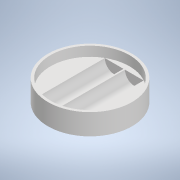
# Autodesk Inventor part: EnclosureBase
Saved by Autodesk Inventor 2020 (Build 240168000, 168)
## iProperties
Created: 2020-10-17
Part Number: EnclosureBase
Material: Generic
Document SubType Name: Modeling
Designer: vmiguel
Density: 1 g/cm^3
Appearance: Default
Author: vmiguel
Autodesk Inventor part; units mm, degrees
ref_plane "YZ Plane" through (0, 0, 0) normal (1, 0, 0) x (0, 1, 0)
ref_plane "XZ Plane" through (0, 0, 0) normal (0, 1, 0) x (-1, 0, 0)
ref_plane "XY Plane" through (0, 0, 0) normal (0, 0, 1) x (1, 0, 0)
sketch "Sketch1" plane through (0, 0, 0) normal (0, 1, 0) x (-1, 0, 0)
  circle A0 centre (0, 0) radius 50
  dimension "d0" = 100
  constraints: 1 centre point, 1 coincident
  measures "d0" diameter of A0
extrude "Extrusion1" add sketch "Sketch1" along normal blind 25
sketch "Sketch2" plane through (0, 0, 0) normal (0, -1, 0) x (1, 0, 0)
  circle A0 centre (0, 0) radius 25.25
  dimension "d3" = 50.5
  constraints: 1 centre point, 1 coincident
  measures "d3" diameter of A0
extrude "Extrusion2" cut sketch "Sketch2" against normal blind 0.4
sketch "Sketch3" plane through (0, 25, 0) normal (0, 1, 0) x (1, 0, 0)
  circle A0 centre (0, 0) radius 47
  circle A1 centre (0, 0) radius 50 projected
  dimension "d6" = 3
  constraints: 1 centre point, 1 coincident
  measures "d6" radial gap between concentric circles of A1 A0
extrude "Extrusion3" cut sketch "Sketch3" against normal blind 11.5 contours A0
sketch "Sketch5" plane through (0, 0, 0) normal (0, 0, 1) x (1, 0, 0)
  line L0 (-47, 13.5) -> (47, 13.5) construction
  circle A0 centre (12, 13.5) radius 11.125
  circle A1 centre (-12, 13.5) radius 11.125
  line L1 (0, 30.15) -> (0, -5.025) construction
  point P0 (0, 0)
  dimension "d9" = 22.25
  dimension "d10" = 22.25
  dimension "d11" = 12
  dimension "d12" = 12
  constraints: 2 centre point, 2 point on line
  measures "d9" diameter of A0
  measures "d10" diameter of A1
  measures "d11" distance from line of L1 A0.centre
  measures "d12" distance from line of A1.centre L1
extrude "Extrusion4" cut sketch "Sketch5" against normal mid plane 81.5
sketch "Sketch6" plane through (0, 0, 0) normal (0, -1, 0) x (1, 0, 0)
  line L0 (-30.5879, 38.6446) -> (30.5879, 38.6446) construction
  line L1 (30.5879, 38.6446) -> (30.5879, 30) construction
  line L2 (30.5879, 30) -> (-30.5879, 30) construction
  line L3 (-30.5879, 30) -> (-30.5879, 38.6446) construction
  circle A0 centre (0, 0) radius 25.25 projected
  spline S0 degree 2 poles (-20.901, 30.524) (-20.0192, 31.1693) (-19.1182, 33.8658) knots 0 0 0 1 1 1
  spline S1 degree 2 poles (-19.1182, 33.8658) (-18.6006, 35.4313) (-18.3962, 36.6965) knots 0 0 0 1 1 1
  spline S2 degree 2 poles (-18.3962, 36.6965) (-18.3387, 37.0479) (-18.3387, 37.2396) knots 0 0 0 1 1 1
  spline S3 degree 2 poles (-18.3387, 37.2396) (-18.5495, 37.2268) (-18.7284, 37.1246) knots 0 0 0 1 1 1
  line L4 (-18.7284, 37.1246) -> (-19.1118, 36.9073)
  spline S4 degree 2 poles (-19.1118, 36.9073) (-19.2652, 36.8179) (-19.7955, 37.2652) (-19.7508, 37.5783) (-19.4441, 37.7764) (-19.246, 37.853) knots 0 0 0 1 2 3 4 4 4
  spline S5 degree 2 poles (-19.246, 37.853) (-18.8307, 38) (-18.262, 38) (-17.8275, 37.9105) (-17.6486, 37.8083) knots 0 0 0 1 2 3 3 3
  spline S6 degree 2 poles (-17.6486, 37.8083) (-17.2396, 37.5719) (-17.2268, 37.1374) knots 0 0 0 1 1 1
  spline S7 degree 2 poles (-17.2268, 37.1374) (-17.2077, 36.3706) (-17.7444, 34.5495) knots 0 0 0 1 1 1
  spline S8 degree 2 poles (-17.7444, 34.5495) (-18.5942, 31.6613) (-19.738, 30.492) knots 0 0 0 1 1 1
  spline S9 degree 2 poles (-19.738, 30.492) (-20.0511, 30.1661) (-20.3898, 30.0511) knots 0 0 0 1 1 1
  spline S10 degree 2 poles (-20.3898, 30.0511) (-20.4792, 30.0128) (-20.6709, 30.0128) (-20.8243, 30.0831) (-20.8754, 30.1342) knots 0 0 0 1 2 3 3 3
  spline S11 degree 2 poles (-20.8754, 30.1342) (-20.9776, 30.23) (-20.9776, 30.4665) (-20.901, 30.524) knots 0 0 0 1 2 2 2
  spline S12 degree 2 poles (-13.6358, 30.8051) (-13.7444, 31.0927) (-13.7188, 31.9042) (-13.5144, 33.0479) (-13.2971, 33.7061) knots 0 0 0 1 2 3 3 3
  spline S13 degree 2 poles (-13.2971, 33.7061) (-12.7987, 35.2204) (-11.9489, 36.3898) knots 0 0 0 1 1 1
  spline S14 degree 2 poles (-11.9489, 36.3898) (-11.8019, 36.5879) (-11.476, 36.5879) (-11.1693, 36.4473) (-11.0479, 36.345) knots 0 0 0 1 2 3 3 3
  spline S15 degree 2 poles (-11.0479, 36.345) (-10.754, 36.1022) (-10.8562, 35.9489) knots 0 0 0 1 1 1
  spline S16 degree 2 poles (-10.8562, 35.9489) (-11.5719, 34.7923) (-12.0319, 33.8658) knots 0 0 0 1 1 1
  spline S17 degree 2 poles (-12.0319, 33.8658) (-10.8754, 33.9425) (-9.9936, 34.6006) knots 0 0 0 1 1 1
  spline S18 degree 2 poles (-9.9936, 34.6006) (-9.0224, 35.3099) (-9.0224, 36.3259) knots 0 0 0 1 1 1
  spline S19 degree 2 poles (-9.0224, 36.3259) (-9.0224, 37.016) (-9.7125, 37.2077) knots 0 0 0 1 1 1
  spline S20 degree 2 poles (-9.7125, 37.2077) (-9.9169, 37.2652) (-10.4984, 37.2652) (-11.1182, 37.1438) (-11.3994, 37.0415) knots 0 0 0 1 2 3 3 3
  spline S21 degree 2 poles (-11.3994, 37.0415) (-11.9681, 36.8307) (-12.4409, 36.492) knots 0 0 0 1 1 1
  spline S22 degree 2 poles (-12.4409, 36.492) (-12.5687, 36.3962) (-12.7987, 36.3962) (-13.0607, 36.5112) (-13.1629, 36.6006) knots 0 0 0 1 2 3 3 3
  spline S23 degree 2 poles (-13.1629, 36.6006) (-13.5655, 36.9329) (-13.0543, 37.2971) knots 0 0 0 1 1 1
  spline S24 degree 2 poles (-13.0543, 37.2971) (-12.3131, 37.8211) (-10.8626, 37.9744) knots 0 0 0 1 1 1
  spline S25 degree 2 poles (-10.8626, 37.9744) (-10.5942, 38) (-9.6869, 38) (-8.7412, 37.6997) (-8.4601, 37.4505) knots 0 0 0 1 2 3 3 3
  spline S26 degree 2 poles (-8.4601, 37.4505) (-7.9297, 36.984) (-7.9297, 36.1406) knots 0 0 0 1 1 1
  spline S27 degree 2 poles (-7.9297, 36.1406) (-7.9297, 35.3866) (-8.5304, 34.6518) knots 0 0 0 1 1 1
  spline S28 degree 2 poles (-8.5304, 34.6518) (-9.0735, 33.9681) (-9.9425, 33.5463) knots 0 0 0 1 1 1
  spline S29 degree 2 poles (-9.9425, 33.5463) (-9.5272, 33.361) (-9.1118, 32.7029) (-9.131, 31.9425) (-9.4121, 31.3035) (-9.8914, 30.7859) (-10.5176, 30.3962) (-10.8626, 30.2684) knots 0 0 0 1 2 3 4 5 6 6 6
  spline S30 degree 2 poles (-10.8626, 30.2684) (-11.5719, 30) (-12.3067, 30) knots 0 0 0 1 1 1
  spline S31 degree 2 poles (-12.3067, 30) (-13.3355, 30) (-13.6358, 30.8051) knots 0 0 0 1 1 1
  spline S32 degree 2 poles (-12.3962, 33.0351) (-12.7859, 32.0703) (-12.8051, 31.3546) knots 0 0 0 1 1 1
  spline S33 degree 2 poles (-12.8051, 31.3546) (-12.8179, 31.0096) (-12.4537, 30.6326) (-11.8211, 30.6326) (-11.1438, 30.9073) (-10.8626, 31.1438) knots 0 0 0 1 2 3 4 4 4
  spline S34 degree 2 poles (-10.8626, 31.1438) (-10.2236, 31.6869) (-10.1981, 32.3706) knots 0 0 0 1 1 1
  spline S35 degree 2 poles (-10.1981, 32.3706) (-10.1853, 32.9968) (-10.7604, 33.2204) knots 0 0 0 1 1 1
  spline S36 degree 2 poles (-10.7604, 33.2204) (-10.9393, 33.2843) (-11.1374, 33.3035) knots 0 0 0 1 1 1
  spline S37 degree 2 poles (-11.1374, 33.3035) (-11.3738, 33.2971) (-12.2364, 33.0735) (-12.3962, 33.0351) knots 0 0 0 1 2 2 2
  spline S38 degree 2 poles (-8.0192, 31.8403) (-8, 32.2875) (-7.7444, 33.099) (-7.3163, 33.8594) (-6.7412, 34.5367) (-6.4026, 34.7923) knots 0 0 0 1 2 3 4 4 4
  spline S39 degree 2 poles (-6.4026, 34.7923) (-5.6677, 35.3419) (-4.9265, 35.3419) knots 0 0 0 1 1 1
  spline S40 degree 2 poles (-4.9265, 35.3419) (-4.0511, 35.3419) (-3.7572, 34.6198) knots 0 0 0 1 1 1
  spline S41 degree 2 poles (-3.7572, 34.6198) (-3.655, 34.377) (-3.6677, 33.7061) (-3.9105, 33.1374) (-4.345, 32.6709) (-4.9457, 32.3067) (-5.2971, 32.1789) knots 0 0 0 1 2 3 4 5 5 5
  spline S42 degree 2 poles (-5.2971, 32.1789) (-6.0256, 31.9233) (-6.8498, 31.9105) knots 0 0 0 1 1 1
  spline S43 degree 2 poles (-6.8498, 31.9105) (-6.869, 31.8403) (-6.8818, 31.5527) (-6.8115, 31.2013) (-6.722, 31.0607) knots 0 0 0 1 2 3 3 3
  spline S44 degree 2 poles (-6.722, 31.0607) (-6.5367, 30.754) (-6.1917, 30.754) knots 0 0 0 1 1 1
  spline S45 degree 2 poles (-6.1917, 30.754) (-5.5974, 30.754) (-5.0351, 31.1054) knots 0 0 0 1 1 1
  spline S46 degree 2 poles (-5.0351, 31.1054) (-4.8371, 31.2204) (-4.5879, 31.4696) (-4.4026, 31.4696) (-4.2684, 31.2524) (-4.2684, 31.1118) knots 0 0 0 1 2 3 4 4 4
  spline S47 degree 2 poles (-4.2684, 31.1118) (-4.2684, 30.8435) (-4.4217, 30.6454) knots 0 0 0 1 1 1
  spline S48 degree 2 poles (-4.4217, 30.6454) (-5.0607, 30) (-6.3323, 30) knots 0 0 0 1 1 1
  spline S49 degree 2 poles (-6.3323, 30) (-7.0863, 30) (-7.5399, 30.4473) knots 0 0 0 1 1 1
  spline S50 degree 2 poles (-7.5399, 30.4473) (-8.0511, 30.9585) (-8.0192, 31.8403) knots 0 0 0 1 1 1
  spline S51 degree 2 poles (-5.0351, 34.6581) (-5.5719, 34.6581) (-6.0703, 33.9233) knots 0 0 0 1 1 1
  spline S52 degree 2 poles (-6.0703, 33.9233) (-6.4856, 33.2907) (-6.7412, 32.4217) knots 0 0 0 1 1 1
  spline S53 degree 2 poles (-6.7412, 32.4217) (-5.8914, 32.5112) (-5.2652, 33.099) knots 0 0 0 1 1 1
  spline S54 degree 2 poles (-5.2652, 33.099) (-4.6837, 33.6486) (-4.6837, 34.6581) (-5.0351, 34.6581) knots 0 0 0 1 2 2 2
  spline S55 degree 2 poles (-2.8818, 30.2556) (-3.0096, 30.3898) (-3.1693, 30.8051) (-3.1693, 31.3482) (-2.9201, 32.2684) (-2.722, 32.8562) knots 0 0 0 1 2 3 4 4 4
  line L5 (-2.722, 32.8562) -> (-2.2939, 34.1278)
  spline S56 degree 2 poles (-2.2939, 34.1278) (-1.3802, 36.7859) (-1.2396, 38.2364) knots 0 0 0 1 1 1
  spline S57 degree 2 poles (-1.2396, 38.2364) (-1.1885, 38.6645) (-0.8179, 38.6645) knots 0 0 0 1 1 1
  spline S58 degree 2 poles (-0.8179, 38.6645) (-0.5815, 38.6645) (-0.4281, 38.5559) knots 0 0 0 1 1 1
  spline S59 degree 2 poles (-0.4281, 38.5559) (-0.1342, 38.3323) (-0.1534, 37.7764) (-0.3259, 36.984) (-0.607, 36.0511) (-0.7796, 35.5272) knots 0 0 0 1 2 3 4 4 4
  line L6 (-0.7796, 35.5272) -> (-1.4888, 33.4569)
  spline S60 degree 2 poles (-1.4888, 33.4569) (-2.0958, 31.6869) (-2.0958, 31.1693) knots 0 0 0 1 1 1
  spline S61 degree 2 poles (-2.0958, 31.1693) (-2.0958, 30.8946) (-1.8722, 30.8946) knots 0 0 0 1 1 1
  spline S62 degree 2 poles (-1.8722, 30.8946) (-1.655, 30.8946) (-1.3035, 31.0799) (-1.2524, 31.0799) knots 0 0 0 1 2 2 2
  spline S63 degree 2 poles (-1.2524, 31.0799) (-1.1438, 31.0799) (-1.1438, 30.9712) knots 0 0 0 1 1 1
  spline S64 degree 2 poles (-1.1438, 30.9712) (-1.1438, 30.5176) (-1.6102, 30.2109) knots 0 0 0 1 1 1
  spline S65 degree 2 poles (-1.6102, 30.2109) (-1.9233, 30) (-2.4409, 30) (-2.754, 30.1214) (-2.8818, 30.2556) knots 0 0 0 1 2 3 3 3
  spline S66 degree 2 poles (1.508, 31.0096) (1.6358, 31.0096) (1.6358, 30.8307) knots 0 0 0 1 1 1
  spline S67 degree 2 poles (1.6358, 30.8307) (1.6358, 30.6006) (1.4313, 30.3578) knots 0 0 0 1 1 1
  spline S68 degree 2 poles (1.4313, 30.3578) (1.1246, 30) (0.607, 30) knots 0 0 0 1 1 1
  spline S69 degree 2 poles (0.607, 30) (0.0128, 30) (-0.2045, 30.4792) knots 0 0 0 1 1 1
  spline S70 degree 2 poles (-0.2045, 30.4792) (-0.2875, 30.6518) (-0.2875, 31.131) (-0.1214, 31.7188) (0.1278, 32.3642) (0.2812, 32.6965) knots 0 0 0 1 2 3 4 4 4
  line L7 (0.2812, 32.6965) -> (0.5495, 33.3419)
  spline S71 degree 2 poles (0.5495, 33.3419) (0.8435, 34.0639) (0.8435, 34.524) (0.7476, 34.6709) (0.6901, 34.7093) knots 0 0 0 1 2 3 3 3
  line L8 (0.6901, 34.7093) -> (0.5879, 34.7859)
  spline S72 degree 2 poles (0.5879, 34.7859) (0.5367, 34.8179) (0.5367, 34.9968) (0.6773, 35.1629) (0.7923, 35.2204) knots 0 0 0 1 2 3 3 3
  spline S73 degree 2 poles (0.7923, 35.2204) (1.0224, 35.3419) (1.3291, 35.3419) knots 0 0 0 1 1 1
  spline S74 degree 2 poles (1.3291, 35.3419) (2.0767, 35.3419) (2.0767, 34.9457) knots 0 0 0 1 1 1
  spline S75 degree 2 poles (2.0767, 34.9457) (2.0767, 34.4856) (1.5974, 33.3035) (1.4313, 32.9457) knots 0 0 0 1 2 2 2
  line L9 (1.4313, 32.9457) -> (1.1246, 32.2364)
  spline S76 degree 2 poles (1.1246, 32.2364) (0.7859, 31.4633) (0.7859, 31.1182) knots 0 0 0 1 1 1
  spline S77 degree 2 poles (0.7859, 31.1182) (0.7859, 30.8946) (1.0096, 30.8946) knots 0 0 0 1 1 1
  spline S78 degree 2 poles (1.0096, 30.8946) (1.2268, 30.8946) (1.4569, 31.0096) (1.508, 31.0096) knots 0 0 0 1 2 2 2
  spline S79 degree 2 poles (2.5495, 36.5367) (2.4409, 36.4217) (2.1534, 36.2684) (1.8403, 36.2364) (1.5591, 36.3706) (1.4569, 36.492) knots 0 0 0 1 2 3 4 4 4
  spline S80 degree 2 poles (1.4569, 36.492) (1.2332, 36.7476) (1.2332, 37.2652) (1.4058, 37.5272) (1.5335, 37.6102) knots 0 0 0 1 2 3 3 3
  spline S81 degree 2 poles (1.5335, 37.6102) (1.7764, 37.77) (2.2109, 37.77) (2.4473, 37.7061) (2.5495, 37.6358) knots 0 0 0 1 2 3 3 3
  spline S82 degree 2 poles (2.5495, 37.6358) (2.8051, 37.4696) (2.8051, 36.984) (2.6645, 36.6581) (2.5495, 36.5367) knots 0 0 0 1 2 3 3 3
  spline S83 degree 2 poles (2.8435, 31.8403) (2.8626, 32.2875) (3.1182, 33.099) (3.5463, 33.8594) (4.1214, 34.5367) (4.4601, 34.7923) knots 0 0 0 1 2 3 4 4 4
  spline S84 degree 2 poles (4.4601, 34.7923) (5.1949, 35.3419) (5.9361, 35.3419) knots 0 0 0 1 1 1
  spline S85 degree 2 poles (5.9361, 35.3419) (6.8115, 35.3419) (7.1054, 34.6198) knots 0 0 0 1 1 1
  spline S86 degree 2 poles (7.1054, 34.6198) (7.2077, 34.377) (7.1949, 33.7061) (6.9521, 33.1374) (6.5176, 32.6709) (5.9169, 32.3067) (5.5655, 32.1789) knots 0 0 0 1 2 3 4 5 5 5
  spline S87 degree 2 poles (5.5655, 32.1789) (4.8371, 31.9233) (4.0128, 31.9105) knots 0 0 0 1 1 1
  spline S88 degree 2 poles (4.0128, 31.9105) (3.9936, 31.8403) (3.9808, 31.5527) (4.0511, 31.2013) (4.1406, 31.0607) knots 0 0 0 1 2 3 3 3
  spline S89 degree 2 poles (4.1406, 31.0607) (4.3259, 30.754) (4.6709, 30.754) knots 0 0 0 1 1 1
  spline S90 degree 2 poles (4.6709, 30.754) (5.2652, 30.754) (5.8275, 31.1054) knots 0 0 0 1 1 1
  spline S91 degree 2 poles (5.8275, 31.1054) (6.0256, 31.2204) (6.2748, 31.4696) (6.4601, 31.4696) (6.5942, 31.2524) (6.5942, 31.1118) knots 0 0 0 1 2 3 4 4 4
  spline S92 degree 2 poles (6.5942, 31.1118) (6.5942, 30.8435) (6.4409, 30.6454) knots 0 0 0 1 1 1
  spline S93 degree 2 poles (6.4409, 30.6454) (5.8019, 30) (4.5304, 30) knots 0 0 0 1 1 1
  spline S94 degree 2 poles (4.5304, 30) (3.7764, 30) (3.3227, 30.4473) knots 0 0 0 1 1 1
  spline S95 degree 2 poles (3.3227, 30.4473) (2.8115, 30.9585) (2.8435, 31.8403) knots 0 0 0 1 1 1
  spline S96 degree 2 poles (5.8275, 34.6581) (5.2907, 34.6581) (4.7923, 33.9233) knots 0 0 0 1 1 1
  spline S97 degree 2 poles (4.7923, 33.9233) (4.377, 33.2907) (4.1214, 32.4217) knots 0 0 0 1 1 1
  spline S98 degree 2 poles (4.1214, 32.4217) (4.9712, 32.5112) (5.5974, 33.099) knots 0 0 0 1 1 1
  spline S99 degree 2 poles (5.5974, 33.099) (6.1789, 33.6486) (6.1789, 34.6581) (5.8275, 34.6581) knots 0 0 0 1 2 2 2
  spline S100 degree 2 poles (7.7508, 30.5495) (7.6741, 30.7157) (7.6741, 31.1757) (7.8147, 31.7316) (8.0383, 32.3131) (8.1789, 32.6198) knots 0 0 0 1 2 3 4 4 4
  line L10 (8.1789, 32.6198) -> (8.4409, 33.2077)
  spline S101 degree 2 poles (8.4409, 33.2077) (8.9457, 34.377) (8.8115, 34.5879) knots 0 0 0 1 1 1
  spline S102 degree 2 poles (8.8115, 34.5879) (8.754, 34.6837) (8.5751, 34.7859) knots 0 0 0 1 1 1
  spline S103 degree 2 poles (8.5751, 34.7859) (8.524, 34.8179) (8.524, 34.9968) (8.6709, 35.1629) (8.7923, 35.2204) knots 0 0 0 1 2 3 3 3
  spline S104 degree 2 poles (8.7923, 35.2204) (9.0351, 35.3419) (9.5399, 35.3419) (9.8019, 35.2332) (9.885, 35.1502) knots 0 0 0 1 2 3 3 3
  spline S105 degree 2 poles (9.885, 35.1502) (10.0511, 34.984) (10.0511, 34.5048) (9.8658, 33.8978) (9.5911, 33.2332) (9.4249, 32.8882) knots 0 0 0 1 2 3 4 4 4
  line L11 (9.4249, 32.8882) -> (9.1246, 32.2173)
  spline S106 degree 2 poles (9.1246, 32.2173) (8.8051, 31.476) (8.8051, 31.2396) knots 0 0 0 1 1 1
  spline S107 degree 2 poles (8.8051, 31.2396) (8.8051, 30.7668) (9.1374, 30.7668) knots 0 0 0 1 1 1
  spline S108 degree 2 poles (9.1374, 30.7668) (9.9872, 30.7668) (10.7348, 31.7764) knots 0 0 0 1 1 1
  spline S109 degree 2 poles (10.7348, 31.7764) (11.1693, 32.3642) (11.3546, 33.0543) knots 0 0 0 1 1 1
  spline S110 degree 2 poles (11.3546, 33.0543) (11.4441, 33.3802) (11.4441, 33.9169) (11.4058, 34.2748) (11.3674, 34.4153) knots 0 0 0 1 2 3 3 3
  spline S111 degree 2 poles (11.3674, 34.4153) (11.3035, 34.6581) (11.1438, 34.8371) knots 0 0 0 1 1 1
  spline S112 degree 2 poles (11.1438, 34.8371) (11.0351, 34.9712) (11.2396, 35.1502) knots 0 0 0 1 1 1
  spline S113 degree 2 poles (11.2396, 35.1502) (11.4633, 35.3419) (11.8786, 35.3419) knots 0 0 0 1 1 1
  spline S114 degree 2 poles (11.8786, 35.3419) (12.1342, 35.3419) (12.3259, 35.099) knots 0 0 0 1 1 1
  spline S115 degree 2 poles (12.3259, 35.099) (12.5751, 34.8115) (12.5751, 33.7444) (12.2556, 32.722) (11.7061, 31.7764) (10.9521, 30.9585) (10.5176, 30.6518) knots 0 0 0 1 2 3 4 5 5 5
  spline S116 degree 2 poles (10.5176, 30.6518) (9.5911, 30) (8.6581, 30) knots 0 0 0 1 1 1
  spline S117 degree 2 poles (8.6581, 30) (7.9872, 30) (7.7508, 30.5495) knots 0 0 0 1 1 1
  spline S118 degree 2 poles (13.131, 31.8403) (13.1502, 32.2875) (13.4058, 33.099) (13.8339, 33.8594) (14.4089, 34.5367) (14.7476, 34.7923) knots 0 0 0 1 2 3 4 4 4
  spline S119 degree 2 poles (14.7476, 34.7923) (15.4824, 35.3419) (16.2236, 35.3419) knots 0 0 0 1 1 1
  spline S120 degree 2 poles (16.2236, 35.3419) (17.099, 35.3419) (17.393, 34.6198) knots 0 0 0 1 1 1
  spline S121 degree 2 poles (17.393, 34.6198) (17.4952, 34.377) (17.4824, 33.7061) (17.2396, 33.1374) (16.8051, 32.6709) (16.2045, 32.3067) (15.853, 32.1789) knots 0 0 0 1 2 3 4 5 5 5
  spline S122 degree 2 poles (15.853, 32.1789) (15.1246, 31.9233) (14.3003, 31.9105) knots 0 0 0 1 1 1
  spline S123 degree 2 poles (14.3003, 31.9105) (14.2812, 31.8403) (14.2684, 31.5527) (14.3387, 31.2013) (14.4281, 31.0607) knots 0 0 0 1 2 3 3 3
  spline S124 degree 2 poles (14.4281, 31.0607) (14.6134, 30.754) (14.9585, 30.754) knots 0 0 0 1 1 1
  spline S125 degree 2 poles (14.9585, 30.754) (15.5527, 30.754) (16.115, 31.1054) knots 0 0 0 1 1 1
  spline S126 degree 2 poles (16.115, 31.1054) (16.3131, 31.2204) (16.5623, 31.4696) (16.7476, 31.4696) (16.8818, 31.2524) (16.8818, 31.1118) knots 0 0 0 1 2 3 4 4 4
  spline S127 degree 2 poles (16.8818, 31.1118) (16.8818, 30.8435) (16.7284, 30.6454) knots 0 0 0 1 1 1
  spline S128 degree 2 poles (16.7284, 30.6454) (16.0895, 30) (14.8179, 30) knots 0 0 0 1 1 1
  spline S129 degree 2 poles (14.8179, 30) (14.0639, 30) (13.6102, 30.4473) knots 0 0 0 1 1 1
  spline S130 degree 2 poles (13.6102, 30.4473) (13.099, 30.9585) (13.131, 31.8403) knots 0 0 0 1 1 1
  spline S131 degree 2 poles (16.115, 34.6581) (15.5783, 34.6581) (15.0799, 33.9233) knots 0 0 0 1 1 1
  spline S132 degree 2 poles (15.0799, 33.9233) (14.6645, 33.2907) (14.4089, 32.4217) knots 0 0 0 1 1 1
  spline S133 degree 2 poles (14.4089, 32.4217) (15.2588, 32.5112) (15.885, 33.099) knots 0 0 0 1 1 1
  spline S134 degree 2 poles (15.885, 33.099) (16.4665, 33.6486) (16.4665, 34.6581) (16.115, 34.6581) knots 0 0 0 1 2 2 2
  point P0 (0, 30)
  dimension "d17" = 30
  constraints: 1 midpoint, 1 vertical alignment, 2 other
  measures "d17" distance from line of point (0, 0) L2
emboss "Emboss1" sketch "Sketch6" operation cut depth 1.5 direction (0, 1, 0) contours S0 S1 S2 S3 L4 S4 S5 S6 S7 S8 S9 S10 S11 | S12 S13 S14 S15 S16 S17 S18 S19 S20 S21 S22 S23 S24 S25 S26 S27 S28 S29 S30 S31 | S38 S39 S40 S41 S42 S43 S44 S45 S46 S47 S48 S49 S50 | S55 L5 S56 S57 S58 S59 L6 S60 S61 S62 S63 S64 S65 | S66 S67 S68 S69 S70 L7 S71 L8 S72 S73 S74 S75 L9 S76 S77 S78 | S79 S80 S81 S82 | S83 S84 S85 S86 S87 S88 S89 S90 S91 S92 S93 S94 S95 | S100 L10 S101 S102 S103 S104 S105 L11 S106 S107 S108 S109 S110 S111 S112 S113 S114 S115 S116 S117 | S118 S119 S120 S121 S122 S123 S124 S125 S126 S127 S128 S129 S130
sketch "Sketch7" plane through (0, 13.5, 0) normal (0, 1, 0) x (1, 0, 0)
  line L0 (23.125, -24.5019) -> (23.125, 24.5019) construction
  line L1 (23.125, 24.5019) -> (33.125, 24.5019) construction
  line L2 (33.125, 24.5019) -> (33.125, -24.5019) construction
  line L3 (33.125, -24.5019) -> (23.125, -24.5019) construction
  line L4 (-23.125, -40.75) -> (-23.125, 40.75) projected
  line L5 (-33.125, -20.8949) -> (-33.125, 20.8949) construction
  line L6 (-33.125, 20.8949) -> (-23.125, 20.8949) construction
  line L7 (-23.125, 20.8949) -> (-23.125, -20.8949) construction
  line L8 (-23.125, -20.8949) -> (-33.125, -20.8949) construction
  line L9 (23.125, 40.75) -> (23.125, -40.75) projected
  spline S0 degree 2 poles (-25.387, -7.9808) (-25.6042, -8.0958) (-26.1026, -8.2045) (-26.6522, -8.2045) (-27.5467, -8.0192) (-28.5435, -7.6869) (-29.5851, -7.2524) (-30.0835, -7.0096) knots 0 0 0 1 2 3 4 5 6 6 6
  spline S1 degree 2 poles (-30.0835, -7.0096) (-31.1186, -6.5112) (-31.8726, -6.0128) knots 0 0 0 1 1 1
  line L10 (-31.8726, -6.0128) -> (-31.8726, -6.0703)
  spline S2 degree 2 poles (-31.8726, -6.0703) (-31.8726, -6.6773) (-31.5978, -7.2013) knots 0 0 0 1 1 1
  spline S3 degree 2 poles (-31.5978, -7.2013) (-31.502, -7.3291) (-31.502, -7.4441) knots 0 0 0 1 1 1
  spline S4 degree 2 poles (-31.502, -7.4441) (-31.502, -7.6869) (-31.7384, -7.9169) knots 0 0 0 1 1 1
  spline S5 degree 2 poles (-31.7384, -7.9169) (-32.3007, -8.4537) (-32.6713, -7.2843) knots 0 0 0 1 1 1
  spline S6 degree 2 poles (-32.6713, -7.2843) (-32.8502, -6.7412) (-32.8502, -6.0703) (-32.6394, -5.6613) (-32.4988, -5.5208) knots 0 0 0 1 2 3 3 3
  spline S7 degree 2 poles (-32.4988, -5.5208) (-32.2688, -5.2907) (-31.8343, -5.1054) (-31.502, -5.1054) (-30.9397, -5.3035) (-30.6266, -5.4569) knots 0 0 0 1 2 3 4 4 4
  line L11 (-30.6266, -5.4569) -> (-29.9493, -5.8019)
  spline S8 degree 2 poles (-29.9493, -5.8019) (-29.5978, -5.9872) (-28.8183, -6.3578) (-28.0451, -6.722) (-27.6745, -6.869) knots 0 0 0 1 2 3 3 3
  spline S9 degree 2 poles (-27.6745, -6.869) (-26.8566, -7.1757) (-26.2815, -7.1757) knots 0 0 0 1 1 1
  spline S10 degree 2 poles (-26.2815, -7.1757) (-25.9365, -7.1757) (-25.7065, -7.1118) knots 0 0 0 1 1 1
  spline S11 degree 2 poles (-25.7065, -7.1118) (-26.0643, -6.8882) (-26.4541, -6.5623) knots 0 0 0 1 1 1
  line L12 (-26.4541, -6.5623) -> (-27.2592, -5.8466)
  spline S12 degree 2 poles (-27.2592, -5.8466) (-28.5946, -4.6006) (-29.0355, -4.23) knots 0 0 0 1 1 1
  spline S13 degree 2 poles (-29.0355, -4.23) (-30.0643, -3.3546) (-30.9716, -2.8882) knots 0 0 0 1 1 1
  spline S14 degree 2 poles (-30.9716, -2.8882) (-31.3359, -2.7029) (-31.6298, -2.7029) knots 0 0 0 1 1 1
  spline S15 degree 2 poles (-31.6298, -2.7029) (-32.1793, -2.7029) (-32.4541, -3.0032) knots 0 0 0 1 1 1
  spline S16 degree 2 poles (-32.4541, -3.0032) (-32.5627, -3.1118) (-32.8694, -2.9521) (-32.9461, -2.869) knots 0 0 0 1 2 2 2
  spline S17 degree 2 poles (-32.9461, -2.869) (-33.125, -2.6709) (-33.125, -2.1725) (-32.9205, -1.8211) (-32.7608, -1.7125) knots 0 0 0 1 2 3 3 3
  spline S18 degree 2 poles (-32.7608, -1.7125) (-32.4477, -1.4952) (-31.5276, -1.4952) (-30.4924, -1.8914) (-29.5084, -2.5304) (-28.5819, -3.3419) (-28.1601, -3.7636) knots 0 0 0 1 2 3 4 5 5 5
  line L13 (-28.1601, -3.7636) -> (-26.7033, -5.3099)
  spline S19 degree 2 poles (-26.7033, -5.3099) (-26.0004, -6.0064) (-25.7384, -6.2428) knots 0 0 0 1 1 1
  spline S20 degree 2 poles (-25.7384, -6.2428) (-25.24, -6.6901) (-24.9205, -6.9457) (-24.863, -7.1502) (-24.863, -7.5016) (-25.1697, -7.8658) (-25.387, -7.9808) knots 0 0 0 1 2 3 4 5 5 5
  spline S21 degree 2 poles (-25.8598, -0.8243) (-25.8598, -0.6965) (-25.6809, -0.6965) knots 0 0 0 1 1 1
  spline S22 degree 2 poles (-25.6809, -0.6965) (-25.4509, -0.6965) (-25.2081, -0.901) knots 0 0 0 1 1 1
  spline S23 degree 2 poles (-25.2081, -0.901) (-24.8502, -1.2077) (-24.8502, -1.7252) knots 0 0 0 1 1 1
  spline S24 degree 2 poles (-24.8502, -1.7252) (-24.8502, -2.3195) (-25.3295, -2.5367) knots 0 0 0 1 1 1
  spline S25 degree 2 poles (-25.3295, -2.5367) (-25.502, -2.6198) (-25.9812, -2.6198) (-26.5691, -2.4537) (-27.2145, -2.2045) (-27.5467, -2.0511) knots 0 0 0 1 2 3 4 4 4
  line L14 (-27.5467, -2.0511) -> (-28.1921, -1.7827)
  spline S26 degree 2 poles (-28.1921, -1.7827) (-28.9141, -1.4888) (-29.3742, -1.4888) (-29.5212, -1.5847) (-29.5595, -1.6422) knots 0 0 0 1 2 3 3 3
  line L15 (-29.5595, -1.6422) -> (-29.6362, -1.7444)
  spline S27 degree 2 poles (-29.6362, -1.7444) (-29.6681, -1.7955) (-29.847, -1.7955) (-30.0132, -1.655) (-30.0707, -1.5399) knots 0 0 0 1 2 3 3 3
  spline S28 degree 2 poles (-30.0707, -1.5399) (-30.1921, -1.3099) (-30.1921, -1.0032) knots 0 0 0 1 1 1
  spline S29 degree 2 poles (-30.1921, -1.0032) (-30.1921, -0.2556) (-29.7959, -0.2556) knots 0 0 0 1 1 1
  spline S30 degree 2 poles (-29.7959, -0.2556) (-29.3359, -0.2556) (-28.1538, -0.7348) (-27.7959, -0.901) knots 0 0 0 1 2 2 2
  line L16 (-27.7959, -0.901) -> (-27.0867, -1.2077)
  spline S31 degree 2 poles (-27.0867, -1.2077) (-26.3135, -1.5463) (-25.9685, -1.5463) knots 0 0 0 1 1 1
  spline S32 degree 2 poles (-25.9685, -1.5463) (-25.7448, -1.5463) (-25.7448, -1.3227) knots 0 0 0 1 1 1
  spline S33 degree 2 poles (-25.7448, -1.3227) (-25.7448, -1.1054) (-25.8598, -0.8754) (-25.8598, -0.8243) knots 0 0 0 1 2 2 2
  spline S34 degree 2 poles (-31.387, 0.2173) (-31.272, 0.1086) (-31.1186, -0.1789) (-31.0867, -0.492) (-31.2208, -0.7732) (-31.3423, -0.8754) knots 0 0 0 1 2 3 4 4 4
  spline S35 degree 2 poles (-31.3423, -0.8754) (-31.5978, -1.099) (-32.1154, -1.099) (-32.3774, -0.9265) (-32.4605, -0.7987) knots 0 0 0 1 2 3 3 3
  spline S36 degree 2 poles (-32.4605, -0.7987) (-32.6202, -0.5559) (-32.6202, -0.1214) (-32.5563, 0.115) (-32.486, 0.2173) knots 0 0 0 1 2 3 3 3
  spline S37 degree 2 poles (-32.486, 0.2173) (-32.3199, 0.4728) (-31.8343, 0.4728) (-31.5084, 0.3323) (-31.387, 0.2173) knots 0 0 0 1 2 3 3 3
  spline S38 degree 2 poles (-29.2272, 4.1406) (-29.2272, 3.9808) (-28.6138, 3.3994) (-28.3646, 3.1885) knots 0 0 0 1 2 2 2
  line L17 (-28.3646, 3.1885) -> (-27.847, 2.754)
  line L18 (-27.847, 2.754) -> (-26.78, 1.9169)
  spline S39 degree 2 poles (-26.78, 1.9169) (-26.2177, 1.6166) (-25.8407, 1.4505) knots 0 0 0 1 1 1
  line L19 (-25.8407, 1.4505) -> (-25.2464, 1.1757)
  spline S40 degree 2 poles (-25.2464, 1.1757) (-25.0292, 1.0671) (-24.8502, 0.9073) (-24.8502, 0.639) (-24.9461, 0.3834) (-25.0228, 0.2939) knots 0 0 0 1 2 3 4 4 4
  spline S41 degree 2 poles (-25.0228, 0.2939) (-25.1889, 0.1022) (-25.3806, 0.1022) knots 0 0 0 1 1 1
  spline S42 degree 2 poles (-25.3806, 0.1022) (-25.4573, 0.1022) (-25.6809, 0.2109) knots 0 0 0 1 1 1
  line L20 (-25.6809, 0.2109) -> (-26.0962, 0.4089)
  spline S43 degree 2 poles (-26.0962, 0.4089) (-26.2815, 0.4984) (-26.5691, 0.6198) knots 0 0 0 1 1 1
  line L21 (-26.5691, 0.6198) -> (-27.2656, 0.9073)
  spline S44 degree 2 poles (-27.2656, 0.9073) (-28.7736, 1.508) (-29.2145, 1.508) knots 0 0 0 1 1 1
  spline S45 degree 2 poles (-29.2145, 1.508) (-29.4509, 1.508) (-29.5595, 1.3546) knots 0 0 0 1 1 1
  line L22 (-29.5595, 1.3546) -> (-29.6362, 1.2524)
  spline S46 degree 2 poles (-29.6362, 1.2524) (-29.6681, 1.2013) (-29.847, 1.2013) (-30.0132, 1.3419) (-30.0707, 1.4569) knots 0 0 0 1 2 3 3 3
  spline S47 degree 2 poles (-30.0707, 1.4569) (-30.1921, 1.6869) (-30.1921, 2.147) (-30.0899, 2.4026) (-30.0004, 2.492) knots 0 0 0 1 2 3 3 3
  spline S48 degree 2 poles (-30.0004, 2.492) (-29.8215, 2.6837) (-29.4317, 2.6837) (-29.0419, 2.5815) (-28.6394, 2.4345) (-28.2496, 2.2748) (-28.1026, 2.2045) knots 0 0 0 1 2 3 4 5 5 5
  line L23 (-28.1026, 2.2045) -> (-27.8854, 2.1022)
  spline S49 degree 2 poles (-27.8854, 2.1022) (-27.8023, 2.0639) (-27.8343, 2.0831) knots 0 0 0 1 1 1
  spline S50 degree 2 poles (-27.8343, 2.0831) (-28.6202, 2.6518) (-28.8438, 2.8307) knots 0 0 0 1 1 1
  line L24 (-28.8438, 2.8307) -> (-29.2784, 3.1885)
  spline S51 degree 2 poles (-29.2784, 3.1885) (-29.7384, 3.5783) (-29.8854, 3.8019) knots 0 0 0 1 1 1
  spline S52 degree 2 poles (-29.8854, 3.8019) (-30.1921, 4.262) (-30.1921, 4.7796) (-30.0579, 5.1374) (-29.9365, 5.2716) knots 0 0 0 1 2 3 3 3
  spline S53 degree 2 poles (-29.9365, 5.2716) (-29.6745, 5.5527) (-28.8694, 5.5527) (-27.9876, 5.1821) (-27.4445, 4.9137) (-27.1633, 4.7923) knots 0 0 0 1 2 3 4 4 4
  spline S54 degree 2 poles (-27.1633, 4.7923) (-26.3071, 4.4089) (-25.9173, 4.4089) knots 0 0 0 1 1 1
  spline S55 degree 2 poles (-25.9173, 4.4089) (-25.7448, 4.4089) (-25.7448, 4.6837) knots 0 0 0 1 1 1
  spline S56 degree 2 poles (-25.7448, 4.6837) (-25.7448, 4.901) (-25.9301, 5.2524) (-25.9301, 5.3035) knots 0 0 0 1 2 2 2
  spline S57 degree 2 poles (-25.9301, 5.3035) (-25.9301, 5.4121) (-25.8215, 5.4121) knots 0 0 0 1 1 1
  spline S58 degree 2 poles (-25.8215, 5.4121) (-25.3678, 5.4121) (-25.0611, 4.9457) knots 0 0 0 1 1 1
  spline S59 degree 2 poles (-25.0611, 4.9457) (-24.8502, 4.6326) (-24.8502, 4.1086) (-24.9653, 3.77) (-25.0867, 3.6358) knots 0 0 0 1 2 3 3 3
  spline S60 degree 2 poles (-25.0867, 3.6358) (-25.355, 3.3355) (-25.8407, 3.3355) knots 0 0 0 1 1 1
  spline S61 degree 2 poles (-25.8407, 3.3355) (-26.4349, 3.3355) (-27.3231, 3.7061) knots 0 0 0 1 1 1
  spline S62 degree 2 poles (-27.3231, 3.7061) (-27.9301, 3.9808) (-28.1538, 4.0895) knots 0 0 0 1 1 1
  line L25 (-28.1538, 4.0895) -> (-28.518, 4.262)
  spline S63 degree 2 poles (-28.518, 4.262) (-28.8438, 4.4217) (-29.2272, 4.4217) (-29.2272, 4.1406) knots 0 0 0 1 2 2 2
  spline S64 degree 2 poles (-25.8598, 8.0447) (-25.8598, 8.1725) (-25.6809, 8.1725) knots 0 0 0 1 1 1
  spline S65 degree 2 poles (-25.6809, 8.1725) (-25.4509, 8.1725) (-25.2081, 7.9681) knots 0 0 0 1 1 1
  spline S66 degree 2 poles (-25.2081, 7.9681) (-24.8502, 7.6613) (-24.8502, 7.1438) knots 0 0 0 1 1 1
  spline S67 degree 2 poles (-24.8502, 7.1438) (-24.8502, 6.5495) (-25.3295, 6.3323) knots 0 0 0 1 1 1
  spline S68 degree 2 poles (-25.3295, 6.3323) (-25.502, 6.2492) (-25.9812, 6.2492) (-26.5691, 6.4153) (-27.2145, 6.6645) (-27.5467, 6.8179) knots 0 0 0 1 2 3 4 4 4
  line L26 (-27.5467, 6.8179) -> (-28.1921, 7.0863)
  spline S69 degree 2 poles (-28.1921, 7.0863) (-28.9141, 7.3802) (-29.3742, 7.3802) (-29.5212, 7.2843) (-29.5595, 7.2268) knots 0 0 0 1 2 3 3 3
  line L27 (-29.5595, 7.2268) -> (-29.6362, 7.1246)
  spline S70 degree 2 poles (-29.6362, 7.1246) (-29.6681, 7.0735) (-29.847, 7.0735) (-30.0132, 7.2141) (-30.0707, 7.3291) knots 0 0 0 1 2 3 3 3
  spline S71 degree 2 poles (-30.0707, 7.3291) (-30.1921, 7.5591) (-30.1921, 7.8658) knots 0 0 0 1 1 1
  spline S72 degree 2 poles (-30.1921, 7.8658) (-30.1921, 8.6134) (-29.7959, 8.6134) knots 0 0 0 1 1 1
  spline S73 degree 2 poles (-29.7959, 8.6134) (-29.3359, 8.6134) (-28.1538, 8.1342) (-27.7959, 7.9681) knots 0 0 0 1 2 2 2
  line L28 (-27.7959, 7.9681) -> (-27.0867, 7.6613)
  spline S74 degree 2 poles (-27.0867, 7.6613) (-26.3135, 7.3227) (-25.9685, 7.3227) knots 0 0 0 1 1 1
  spline S75 degree 2 poles (-25.9685, 7.3227) (-25.7448, 7.3227) (-25.7448, 7.5463) knots 0 0 0 1 1 1
  spline S76 degree 2 poles (-25.7448, 7.5463) (-25.7448, 7.7636) (-25.8598, 7.9936) (-25.8598, 8.0447) knots 0 0 0 1 2 2 2
  spline S77 degree 2 poles (-31.387, 9.0863) (-31.272, 8.9776) (-31.1186, 8.6901) (-31.0867, 8.377) (-31.2208, 8.0958) (-31.3423, 7.9936) knots 0 0 0 1 2 3 4 4 4
  spline S78 degree 2 poles (-31.3423, 7.9936) (-31.5978, 7.77) (-32.1154, 7.77) (-32.3774, 7.9425) (-32.4605, 8.0703) knots 0 0 0 1 2 3 3 3
  spline S79 degree 2 poles (-32.4605, 8.0703) (-32.6202, 8.3131) (-32.6202, 8.7476) (-32.5563, 8.984) (-32.486, 9.0863) knots 0 0 0 1 2 3 3 3
  spline S80 degree 2 poles (-32.486, 9.0863) (-32.3199, 9.3419) (-31.8343, 9.3419) (-31.5084, 9.2013) (-31.387, 9.0863) knots 0 0 0 1 2 3 3 3
  spline S81 degree 2 poles (32.3199, -17.5687) (32.0323, -17.6773) (31.2208, -17.6518) (30.0771, -17.4473) (29.4189, -17.23) knots 0 0 0 1 2 3 3 3
  spline S82 degree 2 poles (29.4189, -17.23) (27.9046, -16.7316) (26.7352, -15.8818) knots 0 0 0 1 1 1
  spline S83 degree 2 poles (26.7352, -15.8818) (26.5371, -15.7348) (26.5371, -15.4089) (26.6777, -15.1022) (26.78, -14.9808) knots 0 0 0 1 2 3 3 3
  spline S84 degree 2 poles (26.78, -14.9808) (27.0228, -14.6869) (27.1761, -14.7891) knots 0 0 0 1 1 1
  spline S85 degree 2 poles (27.1761, -14.7891) (28.3327, -15.5048) (29.2592, -15.9649) knots 0 0 0 1 1 1
  spline S86 degree 2 poles (29.2592, -15.9649) (29.1825, -14.8083) (28.5244, -13.9265) knots 0 0 0 1 1 1
  spline S87 degree 2 poles (28.5244, -13.9265) (27.8151, -12.9553) (26.7991, -12.9553) knots 0 0 0 1 1 1
  spline S88 degree 2 poles (26.7991, -12.9553) (26.109, -12.9553) (25.9173, -13.6454) knots 0 0 0 1 1 1
  spline S89 degree 2 poles (25.9173, -13.6454) (25.8598, -13.8498) (25.8598, -14.4313) (25.9812, -15.0511) (26.0835, -15.3323) knots 0 0 0 1 2 3 3 3
  spline S90 degree 2 poles (26.0835, -15.3323) (26.2943, -15.901) (26.633, -16.3738) knots 0 0 0 1 1 1
  spline S91 degree 2 poles (26.633, -16.3738) (26.7288, -16.5016) (26.7288, -16.7316) (26.6138, -16.9936) (26.5244, -17.0958) knots 0 0 0 1 2 3 3 3
  spline S92 degree 2 poles (26.5244, -17.0958) (26.1921, -17.4984) (25.8279, -16.9872) knots 0 0 0 1 1 1
  spline S93 degree 2 poles (25.8279, -16.9872) (25.3039, -16.246) (25.1506, -14.7955) knots 0 0 0 1 1 1
  spline S94 degree 2 poles (25.1506, -14.7955) (25.125, -14.5272) (25.125, -13.6198) (25.4253, -12.6741) (25.6745, -12.393) knots 0 0 0 1 2 3 3 3
  spline S95 degree 2 poles (25.6745, -12.393) (26.141, -11.8626) (26.9844, -11.8626) knots 0 0 0 1 1 1
  spline S96 degree 2 poles (26.9844, -11.8626) (27.7384, -11.8626) (28.4732, -12.4633) knots 0 0 0 1 1 1
  spline S97 degree 2 poles (28.4732, -12.4633) (29.1569, -13.0064) (29.5787, -13.8754) knots 0 0 0 1 1 1
  spline S98 degree 2 poles (29.5787, -13.8754) (29.764, -13.4601) (30.4221, -13.0447) (31.1825, -13.0639) (31.8215, -13.345) (32.3391, -13.8243) (32.7288, -14.4505) (32.8566, -14.7955) knots 0 0 0 1 2 3 4 5 6 6 6
  spline S99 degree 2 poles (32.8566, -14.7955) (33.125, -15.5048) (33.125, -16.2396) knots 0 0 0 1 1 1
  spline S100 degree 2 poles (33.125, -16.2396) (33.125, -17.2684) (32.3199, -17.5687) knots 0 0 0 1 1 1
  spline S101 degree 2 poles (30.0899, -16.3291) (31.0547, -16.7188) (31.7704, -16.738) knots 0 0 0 1 1 1
  spline S102 degree 2 poles (31.7704, -16.738) (32.1154, -16.7508) (32.4924, -16.3866) (32.4924, -15.754) (32.2177, -15.0767) (31.9812, -14.7955) knots 0 0 0 1 2 3 4 4 4
  spline S103 degree 2 poles (31.9812, -14.7955) (31.4381, -14.1565) (30.7544, -14.131) knots 0 0 0 1 1 1
  spline S104 degree 2 poles (30.7544, -14.131) (30.1282, -14.1182) (29.9046, -14.6933) knots 0 0 0 1 1 1
  spline S105 degree 2 poles (29.9046, -14.6933) (29.8407, -14.8722) (29.8215, -15.0703) knots 0 0 0 1 1 1
  spline S106 degree 2 poles (29.8215, -15.0703) (29.8279, -15.3067) (30.0515, -16.1693) (30.0899, -16.3291) knots 0 0 0 1 2 2 2
  spline S107 degree 2 poles (31.2847, -11.9521) (30.8375, -11.9329) (30.026, -11.6773) (29.2656, -11.2492) (28.5883, -10.6741) (28.3327, -10.3355) knots 0 0 0 1 2 3 4 4 4
  spline S108 degree 2 poles (28.3327, -10.3355) (27.7831, -9.6006) (27.7831, -8.8594) knots 0 0 0 1 1 1
  spline S109 degree 2 poles (27.7831, -8.8594) (27.7831, -7.984) (28.5052, -7.6901) knots 0 0 0 1 1 1
  spline S110 degree 2 poles (28.5052, -7.6901) (28.748, -7.5879) (29.4189, -7.6006) (29.9876, -7.8434) (30.4541, -8.278) (30.8183, -8.8786) (30.9461, -9.23) knots 0 0 0 1 2 3 4 5 5 5
  spline S111 degree 2 poles (30.9461, -9.23) (31.2017, -9.9585) (31.2145, -10.7827) knots 0 0 0 1 1 1
  spline S112 degree 2 poles (31.2145, -10.7827) (31.2847, -10.8019) (31.5723, -10.8147) (31.9237, -10.7444) (32.0643, -10.655) knots 0 0 0 1 2 3 3 3
  spline S113 degree 2 poles (32.0643, -10.655) (32.371, -10.4696) (32.371, -10.1246) knots 0 0 0 1 1 1
  spline S114 degree 2 poles (32.371, -10.1246) (32.371, -9.5304) (32.0196, -8.9681) knots 0 0 0 1 1 1
  spline S115 degree 2 poles (32.0196, -8.9681) (31.9046, -8.77) (31.6554, -8.5208) (31.6554, -8.3355) (31.8726, -8.2013) (32.0132, -8.2013) knots 0 0 0 1 2 3 4 4 4
  spline S116 degree 2 poles (32.0132, -8.2013) (32.2815, -8.2013) (32.4796, -8.3546) knots 0 0 0 1 1 1
  spline S117 degree 2 poles (32.4796, -8.3546) (33.125, -8.9936) (33.125, -10.2652) knots 0 0 0 1 1 1
  spline S118 degree 2 poles (33.125, -10.2652) (33.125, -11.0192) (32.6777, -11.4728) knots 0 0 0 1 1 1
  spline S119 degree 2 poles (32.6777, -11.4728) (32.1665, -11.984) (31.2847, -11.9521) knots 0 0 0 1 1 1
  spline S120 degree 2 poles (28.4669, -8.9681) (28.4669, -9.5048) (29.2017, -10.0032) knots 0 0 0 1 1 1
  spline S121 degree 2 poles (29.2017, -10.0032) (29.8343, -10.4185) (30.7033, -10.6741) knots 0 0 0 1 1 1
  spline S122 degree 2 poles (30.7033, -10.6741) (30.6138, -9.8243) (30.026, -9.1981) knots 0 0 0 1 1 1
  spline S123 degree 2 poles (30.026, -9.1981) (29.4764, -8.6166) (28.4669, -8.6166) (28.4669, -8.9681) knots 0 0 0 1 2 2 2
  spline S124 degree 2 poles (32.8694, -6.8147) (32.7352, -6.9425) (32.3199, -7.1022) (31.7768, -7.1022) (30.8566, -6.853) (30.2688, -6.655) knots 0 0 0 1 2 3 4 4 4
  line L29 (30.2688, -6.655) -> (28.9972, -6.2268)
  spline S125 degree 2 poles (28.9972, -6.2268) (26.3391, -5.3131) (24.8886, -5.1725) knots 0 0 0 1 1 1
  spline S126 degree 2 poles (24.8886, -5.1725) (24.4605, -5.1214) (24.4605, -4.7508) knots 0 0 0 1 1 1
  spline S127 degree 2 poles (24.4605, -4.7508) (24.4605, -4.5144) (24.5691, -4.361) knots 0 0 0 1 1 1
  spline S128 degree 2 poles (24.5691, -4.361) (24.7927, -4.0671) (25.3486, -4.0863) (26.141, -4.2588) (27.0739, -4.5399) (27.5978, -4.7125) knots 0 0 0 1 2 3 4 4 4
  line L30 (27.5978, -4.7125) -> (29.6681, -5.4217)
  spline S129 degree 2 poles (29.6681, -5.4217) (31.4381, -6.0288) (31.9557, -6.0288) knots 0 0 0 1 1 1
  spline S130 degree 2 poles (31.9557, -6.0288) (32.2304, -6.0288) (32.2304, -5.8051) knots 0 0 0 1 1 1
  spline S131 degree 2 poles (32.2304, -5.8051) (32.2304, -5.5879) (32.0451, -5.2364) (32.0451, -5.1853) knots 0 0 0 1 2 2 2
  spline S132 degree 2 poles (32.0451, -5.1853) (32.0451, -5.0767) (32.1538, -5.0767) knots 0 0 0 1 1 1
  spline S133 degree 2 poles (32.1538, -5.0767) (32.6074, -5.0767) (32.9141, -5.5431) knots 0 0 0 1 1 1
  spline S134 degree 2 poles (32.9141, -5.5431) (33.125, -5.8562) (33.125, -6.3738) (33.0036, -6.6869) (32.8694, -6.8147) knots 0 0 0 1 2 3 3 3
  spline S135 degree 2 poles (32.1154, -2.4249) (32.1154, -2.2971) (32.2943, -2.2971) knots 0 0 0 1 1 1
  spline S136 degree 2 poles (32.2943, -2.2971) (32.5244, -2.2971) (32.7672, -2.5016) knots 0 0 0 1 1 1
  spline S137 degree 2 poles (32.7672, -2.5016) (33.125, -2.8083) (33.125, -3.3259) knots 0 0 0 1 1 1
  spline S138 degree 2 poles (33.125, -3.3259) (33.125, -3.9201) (32.6458, -4.1374) knots 0 0 0 1 1 1
  spline S139 degree 2 poles (32.6458, -4.1374) (32.4732, -4.2204) (31.994, -4.2204) (31.4062, -4.0543) (30.7608, -3.8051) (30.4285, -3.6518) knots 0 0 0 1 2 3 4 4 4
  line L31 (30.4285, -3.6518) -> (29.7831, -3.3834)
  spline S140 degree 2 poles (29.7831, -3.3834) (29.0611, -3.0895) (28.601, -3.0895) (28.4541, -3.1853) (28.4157, -3.2428) knots 0 0 0 1 2 3 3 3
  line L32 (28.4157, -3.2428) -> (28.3391, -3.345)
  spline S141 degree 2 poles (28.3391, -3.345) (28.3071, -3.3962) (28.1282, -3.3962) (27.9621, -3.2556) (27.9046, -3.1406) knots 0 0 0 1 2 3 3 3
  spline S142 degree 2 poles (27.9046, -3.1406) (27.7831, -2.9105) (27.7831, -2.6038) knots 0 0 0 1 1 1
  spline S143 degree 2 poles (27.7831, -2.6038) (27.7831, -1.8562) (28.1793, -1.8562) knots 0 0 0 1 1 1
  spline S144 degree 2 poles (28.1793, -1.8562) (28.6394, -1.8562) (29.8215, -2.3355) (30.1793, -2.5016) knots 0 0 0 1 2 2 2
  line L33 (30.1793, -2.5016) -> (30.8886, -2.8083)
  spline S145 degree 2 poles (30.8886, -2.8083) (31.6617, -3.147) (32.0068, -3.147) knots 0 0 0 1 1 1
  spline S146 degree 2 poles (32.0068, -3.147) (32.2304, -3.147) (32.2304, -2.9233) knots 0 0 0 1 1 1
  spline S147 degree 2 poles (32.2304, -2.9233) (32.2304, -2.7061) (32.1154, -2.476) (32.1154, -2.4249) knots 0 0 0 1 2 2 2
  spline S148 degree 2 poles (26.5883, -1.3834) (26.7033, -1.492) (26.8566, -1.7796) (26.8886, -2.0927) (26.7544, -2.3738) (26.633, -2.476) knots 0 0 0 1 2 3 4 4 4
  spline S149 degree 2 poles (26.633, -2.476) (26.3774, -2.6997) (25.8598, -2.6997) (25.5978, -2.5272) (25.5148, -2.3994) knots 0 0 0 1 2 3 3 3
  spline S150 degree 2 poles (25.5148, -2.3994) (25.355, -2.1565) (25.355, -1.722) (25.4189, -1.4856) (25.4892, -1.3834) knots 0 0 0 1 2 3 3 3
  spline S151 degree 2 poles (25.4892, -1.3834) (25.6554, -1.1278) (26.141, -1.1278) (26.4669, -1.2684) (26.5883, -1.3834) knots 0 0 0 1 2 3 3 3
  spline S152 degree 2 poles (31.2847, -1.0895) (30.8375, -1.0703) (30.026, -0.8147) (29.2656, -0.3866) (28.5883, 0.1885) (28.3327, 0.5272) knots 0 0 0 1 2 3 4 4 4
  spline S153 degree 2 poles (28.3327, 0.5272) (27.7831, 1.262) (27.7831, 2.0032) knots 0 0 0 1 1 1
  spline S154 degree 2 poles (27.7831, 2.0032) (27.7831, 2.8786) (28.5052, 3.1725) knots 0 0 0 1 1 1
  spline S155 degree 2 poles (28.5052, 3.1725) (28.748, 3.2748) (29.4189, 3.262) (29.9876, 3.0192) (30.4541, 2.5847) (30.8183, 1.984) (30.9461, 1.6326) knots 0 0 0 1 2 3 4 5 5 5
  spline S156 degree 2 poles (30.9461, 1.6326) (31.2017, 0.9042) (31.2145, 0.0799) knots 0 0 0 1 1 1
  spline S157 degree 2 poles (31.2145, 0.0799) (31.2847, 0.0607) (31.5723, 0.0479) (31.9237, 0.1182) (32.0643, 0.2077) knots 0 0 0 1 2 3 3 3
  spline S158 degree 2 poles (32.0643, 0.2077) (32.371, 0.393) (32.371, 0.738) knots 0 0 0 1 1 1
  spline S159 degree 2 poles (32.371, 0.738) (32.371, 1.3323) (32.0196, 1.8946) knots 0 0 0 1 1 1
  spline S160 degree 2 poles (32.0196, 1.8946) (31.9046, 2.0927) (31.6554, 2.3419) (31.6554, 2.5272) (31.8726, 2.6613) (32.0132, 2.6613) knots 0 0 0 1 2 3 4 4 4
  spline S161 degree 2 poles (32.0132, 2.6613) (32.2815, 2.6613) (32.4796, 2.508) knots 0 0 0 1 1 1
  spline S162 degree 2 poles (32.4796, 2.508) (33.125, 1.869) (33.125, 0.5974) knots 0 0 0 1 1 1
  spline S163 degree 2 poles (33.125, 0.5974) (33.125, -0.1565) (32.6777, -0.6102) knots 0 0 0 1 1 1
  spline S164 degree 2 poles (32.6777, -0.6102) (32.1665, -1.1214) (31.2847, -1.0895) knots 0 0 0 1 1 1
  spline S165 degree 2 poles (28.4669, 1.8946) (28.4669, 1.3578) (29.2017, 0.8594) knots 0 0 0 1 1 1
  spline S166 degree 2 poles (29.2017, 0.8594) (29.8343, 0.4441) (30.7033, 0.1885) knots 0 0 0 1 1 1
  spline S167 degree 2 poles (30.7033, 0.1885) (30.6138, 1.0383) (30.026, 1.6645) knots 0 0 0 1 1 1
  spline S168 degree 2 poles (30.026, 1.6645) (29.4764, 2.246) (28.4669, 2.246) (28.4669, 1.8946) knots 0 0 0 1 2 2 2
  spline S169 degree 2 poles (32.5755, 3.8179) (32.4093, 3.7412) (31.9493, 3.7412) (31.3934, 3.8818) (30.8119, 4.1054) (30.5052, 4.246) knots 0 0 0 1 2 3 4 4 4
  line L34 (30.5052, 4.246) -> (29.9173, 4.508)
  spline S170 degree 2 poles (29.9173, 4.508) (28.748, 5.0128) (28.5371, 4.8786) knots 0 0 0 1 1 1
  spline S171 degree 2 poles (28.5371, 4.8786) (28.4413, 4.8211) (28.3391, 4.6422) knots 0 0 0 1 1 1
  spline S172 degree 2 poles (28.3391, 4.6422) (28.3071, 4.5911) (28.1282, 4.5911) (27.9621, 4.738) (27.9046, 4.8594) knots 0 0 0 1 2 3 3 3
  spline S173 degree 2 poles (27.9046, 4.8594) (27.7831, 5.1022) (27.7831, 5.607) (27.8918, 5.869) (27.9748, 5.9521) knots 0 0 0 1 2 3 3 3
  spline S174 degree 2 poles (27.9748, 5.9521) (28.141, 6.1182) (28.6202, 6.1182) (29.2272, 5.9329) (29.8918, 5.6581) (30.2368, 5.492) knots 0 0 0 1 2 3 4 4 4
  line L35 (30.2368, 5.492) -> (30.9077, 5.1917)
  spline S175 degree 2 poles (30.9077, 5.1917) (31.649, 4.8722) (31.8854, 4.8722) knots 0 0 0 1 1 1
  spline S176 degree 2 poles (31.8854, 4.8722) (32.3582, 4.8722) (32.3582, 5.2045) knots 0 0 0 1 1 1
  spline S177 degree 2 poles (32.3582, 5.2045) (32.3582, 6.0543) (31.3486, 6.8019) knots 0 0 0 1 1 1
  spline S178 degree 2 poles (31.3486, 6.8019) (30.7608, 7.2364) (30.0707, 7.4217) knots 0 0 0 1 1 1
  spline S179 degree 2 poles (30.0707, 7.4217) (29.7448, 7.5112) (29.2081, 7.5112) (28.8502, 7.4728) (28.7097, 7.4345) knots 0 0 0 1 2 3 3 3
  spline S180 degree 2 poles (28.7097, 7.4345) (28.4669, 7.3706) (28.2879, 7.2109) knots 0 0 0 1 1 1
  spline S181 degree 2 poles (28.2879, 7.2109) (28.1538, 7.1022) (27.9748, 7.3067) knots 0 0 0 1 1 1
  spline S182 degree 2 poles (27.9748, 7.3067) (27.7831, 7.5304) (27.7831, 7.9457) knots 0 0 0 1 1 1
  spline S183 degree 2 poles (27.7831, 7.9457) (27.7831, 8.2013) (28.026, 8.393) knots 0 0 0 1 1 1
  spline S184 degree 2 poles (28.026, 8.393) (28.3135, 8.6422) (29.3806, 8.6422) (30.403, 8.3227) (31.3486, 7.7732) (32.1665, 7.0192) (32.4732, 6.5847) knots 0 0 0 1 2 3 4 5 5 5
  spline S185 degree 2 poles (32.4732, 6.5847) (33.125, 5.6581) (33.125, 4.7252) knots 0 0 0 1 1 1
  spline S186 degree 2 poles (33.125, 4.7252) (33.125, 4.0543) (32.5755, 3.8179) knots 0 0 0 1 1 1
  spline S187 degree 2 poles (31.2847, 9.1981) (30.8375, 9.2173) (30.026, 9.4728) (29.2656, 9.901) (28.5883, 10.476) (28.3327, 10.8147) knots 0 0 0 1 2 3 4 4 4
  spline S188 degree 2 poles (28.3327, 10.8147) (27.7831, 11.5495) (27.7831, 12.2907) knots 0 0 0 1 1 1
  spline S189 degree 2 poles (27.7831, 12.2907) (27.7831, 13.1661) (28.5052, 13.4601) knots 0 0 0 1 1 1
  spline S190 degree 2 poles (28.5052, 13.4601) (28.748, 13.5623) (29.4189, 13.5495) (29.9876, 13.3067) (30.4541, 12.8722) (30.8183, 12.2716) (30.9461, 11.9201) knots 0 0 0 1 2 3 4 5 5 5
  spline S191 degree 2 poles (30.9461, 11.9201) (31.2017, 11.1917) (31.2145, 10.3674) knots 0 0 0 1 1 1
  spline S192 degree 2 poles (31.2145, 10.3674) (31.2847, 10.3482) (31.5723, 10.3355) (31.9237, 10.4058) (32.0643, 10.4952) knots 0 0 0 1 2 3 3 3
  spline S193 degree 2 poles (32.0643, 10.4952) (32.371, 10.6805) (32.371, 11.0256) knots 0 0 0 1 1 1
  spline S194 degree 2 poles (32.371, 11.0256) (32.371, 11.6198) (32.0196, 12.1821) knots 0 0 0 1 1 1
  spline S195 degree 2 poles (32.0196, 12.1821) (31.9046, 12.3802) (31.6554, 12.6294) (31.6554, 12.8147) (31.8726, 12.9489) (32.0132, 12.9489) knots 0 0 0 1 2 3 4 4 4
  spline S196 degree 2 poles (32.0132, 12.9489) (32.2815, 12.9489) (32.4796, 12.7955) knots 0 0 0 1 1 1
  spline S197 degree 2 poles (32.4796, 12.7955) (33.125, 12.1566) (33.125, 10.885) knots 0 0 0 1 1 1
  spline S198 degree 2 poles (33.125, 10.885) (33.125, 10.131) (32.6777, 9.6773) knots 0 0 0 1 1 1
  spline S199 degree 2 poles (32.6777, 9.6773) (32.1665, 9.1661) (31.2847, 9.1981) knots 0 0 0 1 1 1
  spline S200 degree 2 poles (28.4669, 12.1821) (28.4669, 11.6454) (29.2017, 11.147) knots 0 0 0 1 1 1
  spline S201 degree 2 poles (29.2017, 11.147) (29.8343, 10.7316) (30.7033, 10.476) knots 0 0 0 1 1 1
  spline S202 degree 2 poles (30.7033, 10.476) (30.6138, 11.3259) (30.026, 11.9521) knots 0 0 0 1 1 1
  spline S203 degree 2 poles (30.026, 11.9521) (29.4764, 12.5335) (28.4669, 12.5335) (28.4669, 12.1821) knots 0 0 0 1 2 2 2
  spline S204 degree 2 poles (32.1729, 13.8371) (32.0132, 13.8371) (31.7448, 13.9776) (31.6554, 14.0799) knots 0 0 0 1 2 2 2
  spline S205 degree 2 poles (31.6554, 14.0799) (31.4509, 14.2907) (31.4509, 14.5272) knots 0 0 0 1 1 1
  spline S206 degree 2 poles (31.4509, 14.5272) (31.4509, 14.7316) (31.6617, 14.7316) knots 0 0 0 1 1 1
  spline S207 degree 2 poles (31.6617, 14.7316) (32.1921, 14.7316) (32.403, 15.0831) knots 0 0 0 1 1 1
  spline S208 degree 2 poles (32.403, 15.0831) (32.4796, 15.2109) (32.4796, 15.492) (32.4221, 15.6837) (32.3518, 15.7668) knots 0 0 0 1 2 3 3 3
  spline S209 degree 2 poles (32.3518, 15.7668) (32.2049, 15.9521) (31.7959, 15.9521) (31.4509, 15.7668) (31.2656, 15.6262) knots 0 0 0 1 2 3 3 3
  line L36 (31.2656, 15.6262) -> (30.8566, 15.3387)
  spline S210 degree 2 poles (30.8566, 15.3387) (30.0387, 14.7252) (29.3486, 14.7252) knots 0 0 0 1 1 1
  spline S211 degree 2 poles (29.3486, 14.7252) (28.7736, 14.7252) (28.3135, 15.2109) knots 0 0 0 1 1 1
  spline S212 degree 2 poles (28.3135, 15.2109) (27.7831, 15.7604) (27.7831, 16.623) knots 0 0 0 1 1 1
  spline S213 degree 2 poles (27.7831, 16.623) (27.7831, 17.377) (28.1601, 17.8051) knots 0 0 0 1 1 1
  spline S214 degree 2 poles (28.1601, 17.8051) (28.4605, 18.1502) (28.8502, 18.1502) knots 0 0 0 1 1 1
  spline S215 degree 2 poles (28.8502, 18.1502) (29.2528, 18.1502) (29.4892, 17.8435) knots 0 0 0 1 1 1
  spline S216 degree 2 poles (29.4892, 17.8435) (29.7065, 17.5687) (29.649, 17.2939) knots 0 0 0 1 1 1
  spline S217 degree 2 poles (29.649, 17.2939) (29.6234, 17.1725) (29.4253, 17.0383) (29.1697, 17.1214) (28.895, 17.1214) (28.6585, 17.0192) (28.5755, 16.9297) knots 0 0 0 1 2 3 4 5 5 5
  spline S218 degree 2 poles (28.5755, 16.9297) (28.4093, 16.7508) (28.4093, 16.361) (28.4924, 16.1054) (28.5755, 16.0032) knots 0 0 0 1 2 3 3 3
  spline S219 degree 2 poles (28.5755, 16.0032) (28.7608, 15.8051) (29.2975, 15.8051) (29.6873, 15.9904) (30.0771, 16.2588) (30.4732, 16.5783) (30.6905, 16.7125) knots 0 0 0 1 2 3 4 5 5 5
  spline S220 degree 2 poles (30.6905, 16.7125) (31.2081, 17.032) (31.9876, 17.032) (32.518, 16.7061) (32.7033, 16.4441) knots 0 0 0 1 2 3 3 3
  spline S221 degree 2 poles (32.7033, 16.4441) (33.1186, 15.8882) (33.1186, 15.1981) knots 0 0 0 1 1 1
  spline S222 degree 2 poles (33.1186, 15.1981) (33.1186, 14.5399) (32.8055, 14.1566) knots 0 0 0 1 1 1
  spline S223 degree 2 poles (32.8055, 14.1566) (32.5371, 13.8371) (32.1729, 13.8371) knots 0 0 0 1 1 1
  point P0 (0, 0)
  point P1 (-23.125, 0)
  point P2 (-23.125, 0)
  point P3 (23.125, 0)
  point P4 (23.125, 0)
  dimension "d18" = 10
  dimension "d19" = 10
  constraints: 6 midpoint, 2 coincident, 1 parallel, 4 other
  measures "d18" distance of L8.start L8.end
  measures "d19" distance of L2.end L0.start
emboss "Emboss2" sketch "Sketch7" operation cut depth 1.5 direction (0, -1, 0)
equation "\"d10\" = d9"
equation "\"d12\" = d11"
body "Solid1"
